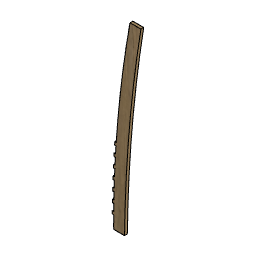
fotur_a (Autodesk Fusion 360 design; units mm, degrees)
Autodesk Fusion 360 part; units mm, degrees
note: some values were not read from the file. Set by a fixed rule: which sketch regions a step uses.
sketch "Sketch1" plane through (0, 0, 0) normal (0, 1, 0) x (1, 0, 0)
  line L0 (0, 0) -> (70, 0)
  arc A0 (70, 0) -> (175, -1200) centre (8172.5, 104.375) ccw
  line L1 (175, -1200) -> (105, -1200)
  arc A1 (0, 0) -> (105, -1200) centre (6634.3619, -24.0871) ccw
  dimension "d3" = 70
  dimension "d9" = 70
  constraint coincident L0.start A1.start
  measures "d3" distance of L0.start L0.end
  measures "d9" distance of A0.end L1.end
extrude "Extrude1" add sketch "Sketch1" along normal blind 18
sketch "Sketch2" plane through (0, 0, 0) normal (0, -1, 0) x (1, 0, 0)
  line L0 (0, 0) -> (70, 0)
  line L1 (0, 15) -> (-9, 15)
  line L2 (-9, 15) -> (-9, 35)
  line L3 (-9, 35) -> (0, 35)
  line L4 (0, 35) -> (45, 35) construction
  line L5 (0.3927, 79.9983) -> (-8.607, 80.0768)
  line L6 (-8.607, 80.0768) -> (-8.4324, 100.0761)
  line L7 (-8.4324, 100.0761) -> (0.5672, 99.9975)
  line L8 (1.0901, 144.9945) -> (-7.9093, 145.0991)
  line L9 (-7.9093, 145.0991) -> (-7.6769, 165.0977)
  line L10 (-7.6769, 165.0977) -> (2.3224, 164.9815)
  line L11 (1.0901, 144.9945) -> (2.3224, 164.9815)
  line L12 (0.3927, 79.9983) -> (0.5672, 99.9975)
  line L13 (1.5567, 164.9815) -> (2.6072, 209.9693)
  line L14 (2.6072, 209.9693) -> (-6.3903, 210.1794)
  line L15 (-6.3903, 210.1794) -> (-5.9235, 230.1739)
  line L16 (-5.9235, 230.1739) -> (3.574, 229.9521)
  line L17 (2.6072, 209.9693) -> (3.574, 229.9521)
  line L18 (4.744, 274.9345) -> (-4.2508, 275.2408)
  line L19 (-4.2508, 275.2408) -> (-3.5702, 295.2292)
  line L20 (-3.5702, 295.2292) -> (5.6245, 294.9161)
  line L21 (4.744, 274.9345) -> (5.6245, 294.9161)
  line L22 (7.492, 339.8725) -> (-1.4992, 340.2687)
  line L23 (-1.4992, 340.2687) -> (-0.6188, 360.2493)
  line L24 (-0.6188, 360.2493) -> (8.5723, 359.8443)
  line L25 (10.9525, 404.7806) -> (1.9659, 405.2718)
  line L26 (1.9659, 405.2718) -> (3.0574, 425.242)
  line L27 (3.0574, 425.242) -> (12.2437, 424.7398)
  line L28 (7.492, 339.8725) -> (8.5723, 359.8443)
  line L29 (10.9525, 404.7806) -> (12.2437, 424.7398)
  line L30 (14.9799, 469.6566) -> (5.9965, 470.2038)
  line L31 (5.9965, 470.2038) -> (7.2126, 490.1668)
  line L32 (7.2126, 490.1668) -> (16.3955, 489.6074)
  line L33 (14.9799, 469.6566) -> (16.3955, 489.6074)
  dimension "d71" = 15
  dimension "d72" = 9
  dimension "d73" = 20
  dimension "d74" = 9
  dimension "d79" = 45
  dimension "d80" = 9
  dimension "d81" = 20
  dimension "d82" = 9
  dimension "d83" = 45
  dimension "d84" = 9
  dimension "d85" = 20
  dimension "d86" = 10
  dimension "d88" = 9
  dimension "d89" = 20
  dimension "d90" = 9.5
  dimension "d92" = 9
  dimension "d93" = 20
  dimension "d94" = 9.2
  dimension "d96" = 9
  dimension "d97" = 20
  dimension "d98" = 9.2
  dimension "d100" = 9
  dimension "d101" = 20
  dimension "d102" = 9.2
  dimension "d103" = 45
  dimension "d104" = 9
  dimension "d105" = 20
  dimension "d106" = 9.2
  constraint perpendicular L1 L2
  constraint horizontal L4
  constraint perpendicular L5 L6
  constraint perpendicular L6 L7
  constraint perpendicular L8 L9
  constraint perpendicular L9 L10
  constraint perpendicular L13 L14
  constraint perpendicular L14 L15
  constraint perpendicular L15 L16
  constraint perpendicular L18 L19
  constraint perpendicular L19 L20
  constraint perpendicular L21 L22
  constraint perpendicular L22 L23
  constraint perpendicular L23 L24
  constraint perpendicular L25 L26
  constraint perpendicular L26 L27
  constraint perpendicular L30 L31
  constraint perpendicular L31 L32
  measures "d71" distance of L0.start L1.start
  measures "d72" distance of L1.start L1.end
  measures "d73" distance of L1.end L2.end
  measures "d74" distance of L2.end L3.end
  measures "d79" distance of L3.end L5.start
  measures "d80" distance of L5.start L5.end
  measures "d81" distance of L5.end L6.end
  measures "d82" distance of L6.end L7.end
  measures "d83" distance of L7.end L8.start
  measures "d84" distance of L8.start L8.end
  measures "d85" distance of L8.end L9.end
  measures "d86" distance of L9.end L10.end
  measures "d88" distance of L13.end L14.end
  measures "d89" distance of L14.end L15.end
  measures "d90" distance of L15.end L16.end
  measures "d92" distance of L18.start L18.end
  measures "d93" distance of L18.end L19.end
  measures "d94" distance of L19.end L20.end
  measures "d96" distance of L22.start L22.end
  measures "d97" distance of L22.end L23.end
  measures "d98" distance of L23.end L24.end
  measures "d100" distance of L25.start L25.end
  measures "d101" distance of L25.end L26.end
  measures "d102" distance of L26.end L27.end
  measures "d103" distance of L27.end L30.start
  measures "d104" distance of L30.start L30.end
  measures "d105" distance of L30.end L31.end
  measures "d106" distance of L31.end L32.end
extrude "Extrude4" add sketch "Sketch2" against normal blind 18
equation "d3 = breidd_fots"
equation "breidd_fots = 70 mm"
equation "haed_fots = 1200 mm"
equation "heildarbreidd = 175 mm"
equation "d9 = breidd_fots"
equation "t = 18 mm"
equation "d11 = t"
equation "nibba_bil = 15 mm"
equation "nibba_breidd = 20 mm"
equation "nibba_lengd = 9 mm"
equation "biti_bil = 15 mm"
equation "plata_þykkt = 50 mm"
equation "bil_fremri_stod = 95 mm"
equation "breidd_fots2 = 90 mm"
equation "bil_support = 50 mm"
equation "d71 = nibba_bil"
equation "d72 = nibba_lengd"
equation "d73 = nibba_breidd"
equation "d74 = nibba_lengd"
equation "d76 = -t"
equation "d79 = 2 * nibba_bil + biti_bil"
equation "d80 = nibba_lengd"
equation "d81 = nibba_breidd"
equation "d82 = nibba_lengd"
equation "d83 = 2 * nibba_bil + biti_bil"
equation "d84 = nibba_lengd"
equation "d85 = nibba_breidd"
equation "d86 = nibba_lengd + 1 mm"
equation "d88 = nibba_lengd"
equation "d89 = nibba_breidd"
equation "d90 = nibba_lengd + 0.5 mm"
equation "d92 = nibba_lengd"
equation "d93 = nibba_breidd"
equation "d94 = nibba_lengd + 0.2 mm"
equation "d96 = nibba_lengd"
equation "d97 = nibba_breidd"
equation "d98 = nibba_lengd + 0.2 mm"
equation "d100 = nibba_lengd"
equation "d101 = nibba_breidd"
equation "d102 = nibba_lengd + 0.2 mm"
equation "d103 = 2 * nibba_bil + biti_bil"
equation "d104 = nibba_lengd"
equation "d105 = nibba_breidd"
equation "d106 = nibba_lengd + 0.2 mm"
